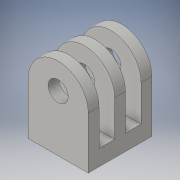
# Autodesk Inventor part: mountBrio
Saved by Autodesk Inventor 2016 (Build 200138000, 138)
## iProperties
Created: 2015-08-22
Part Number: mountBrio
Material: Generic
Document SubType Name: Modeling
Designer: Tyler
Density: 1 g/cm^3
Appearance: Default
Author: Tyler
Autodesk Inventor part; units mm, degrees
ref_plane "YZ Plane" through (0, 0, 0) normal (1, 0, 0) x (0, 1, 0)
ref_plane "XZ Plane" through (0, 0, 0) normal (0, 1, 0) x (-1, 0, 0)
ref_plane "XY Plane" through (0, 0, 0) normal (0, 0, 1) x (1, 0, 0)
sketch "Sketch4" plane through (0, 0, 0) normal (0, 0, 1) x (1, 0, 0)
  line L0 (-10.5, 0) -> (10.5, 0) projected
  line L1 (0, -3.3) -> (0, 19.8) projected
  line L2 (-7.5, 0) -> (7.5, 0)
  line L3 (7.5, 0) -> (7.5, 16.5)
  line L4 (7.5, 16.5) -> (-7.5, 16.5)
  line L5 (-7.5, 16.5) -> (-7.5, 0)
  circle A0 centre (0, 10) radius 2.5
  point P0 (0, 0)
  dimension "d0" = 7.5
  dimension "d1" = 7.5
  dimension "d2" = 16.5
  dimension "d3" = 5
  dimension "d4" = 6.5
  constraints: 8 end point, 2 parallel, 2 point on line, 1 centre point, 1 horizontal, 1 perpendicular
  measures "d0" distance between parallel lines of L1 L5
  measures "d1" distance between parallel lines of L1 L3
  measures "d2" distance between parallel lines of L4 L0
  measures "d3" diameter of A0
  measures "d4" distance from line of L4 A0.centre
extrude "Extrusion1" add sketch "Sketch4" against normal blind 15.9 contours L5 L4 L1 A0 L0 | L1 A0 L4 L3 L0
fillet "Fillet1" radius 7.5 2 edges at (7.5, 16.5, -7.95) (-7.5, 16.5, -7.95)
sketch "Sketch13" plane through (7.5, 9, 0) normal (1, 0, 0) x (0, 0, -1)
  line L0 (0, -12.3) -> (0, 10.8) projected
  line L1 (19.08, -9) -> (-3.18, -9) projected
  line L2 (0, -9) -> (0, 0) projected
  line L3 (0, 7.5) -> (15.9, 7.5) projected
  line L4 (0, -9) -> (2.7, -9)
  line L5 (2.7, -9) -> (2.7, 7.5)
  line L6 (2.7, 7.5) -> (0, 7.5)
  line L7 (0, 7.5) -> (0, -9)
  line L8 (15.9, -9) -> (15.9, 0) projected
  line L9 (15.9, -9) -> (13.2, -9)
  line L10 (13.2, -9) -> (13.2, 7.5)
  line L11 (13.2, 7.5) -> (15.9, 7.5)
  line L12 (15.9, 7.5) -> (15.9, -9)
  line L13 (6.6, -9) -> (9.3, -9)
  line L14 (9.3, -9) -> (9.3, 7.5)
  line L15 (9.3, 7.5) -> (6.6, 7.5)
  line L16 (6.6, 7.5) -> (6.6, -9)
  dimension "d47" = 2.7
  dimension "d48" = 2.7
  dimension "d49" = 2.7
  dimension "d50" = 15.9
  dimension "d51" = 3.9
  dimension "d52" = 3.9
  constraints: 24 end point, 6 parallel, 4 point on line, 3 horizontal, 3 perpendicular
  measures "d47" distance between parallel lines of L5 L0
  measures "d48" distance between parallel lines of L12 L10
  measures "d49" distance between parallel lines of L14 L16
  measures "d50" distance between parallel lines of L12 L0
  measures "d51" distance between parallel lines of L16 L5
  measures "d52" distance between parallel lines of L10 L14
extrude "Extrusion8" cut sketch "Sketch13" against normal through all contours L5 L3 L16 L1 | L14 L3 L10 L1
sketch "Sketch14" plane through (-7.5, 0, -6.6) normal (0, -1, 0) x (1, 0, 0)
  line L0 (0, 6.6) -> (15, 6.6) projected
  line L1 (15, -9.3) -> (0, -9.3) projected
  line L2 (15, 6.6) -> (0, 6.6)
  line L3 (0, 6.6) -> (0, -9.3)
  line L4 (0, -9.3) -> (15, -9.3)
  line L5 (15, -9.3) -> (15, 6.6)
  point P0 (7.5, 6.6)
  constraints: 8 end point, 2 parallel, 1 horizontal, 1 perpendicular
extrude "Extrusion9" add sketch "Sketch14" along normal blind 4
body "Solid1"
